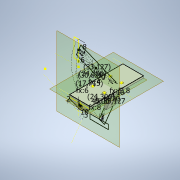
# Autodesk Inventor part: Capping_RotationAnchor
Saved by Autodesk Inventor 2022 (Build 260153000, 153)
## iProperties
Created: 2024-05-05
Part Number: Capping_RotationAnchor
Material: Generic
Document SubType Name: Modeling
Designer: raphael.hauk
Density: 1 g/cm^3
Appearance: Default
Author: raphael.hauk
Autodesk Inventor part; units mm, degrees
ref_plane "YZ Plane" through (0, 0, 0) normal (1, 0, 0) x (0, 1, 0)
ref_plane "XZ Plane" through (0, 0, 0) normal (0, 1, 0) x (-1, 0, 0)
ref_plane "XY Plane" through (0, 0, 0) normal (0, 0, 1) x (1, 0, 0)
sketch "Sketch1" plane through (0, 0, 0) normal (0, 0, 1) x (1, 0, 0)
  line L0 (0, 8) -> (0, -8) projected
  line L1 (0, 8) -> (-4, 8) projected
  line L2 (-4, -8) -> (-4, 8) projected
  line L3 (0, -8) -> (-4, -8) projected
  point P0 (0, 0)
  point P1 (21.25, -8.826)
  constraints: 1 other
sketch "Sketch2" plane through (0, 0, 0) normal (0, 0, 1) x (1, 0, 0)
  line L0 (10, -43.252) -> (26, -43.252)
  line L1 (26, -43.252) -> (26, -47.252)
  line L2 (26, -47.252) -> (10, -47.252)
  line L3 (10, -47.252) -> (10, -43.252)
  line L4 (-4, -8) -> (-4, 8) construction
  line L5 (0, 8) -> (-4, 8) construction
  line L6 (0, 8) -> (0, -8) construction
  line L7 (0, -8) -> (-4, -8) construction
  line L8 (30.626, -12.626) -> (0, 0) construction
  line L9 (18, -43.252) -> (30.626, -12.626) construction
  arc A0 (0, 8) -> (10, -43.252) centre (30.626, -12.626) ccw construction
  line L10 (21.25, -8.826) -> (0, -8.826) construction
  line L11 (1.9057, 4.6226) -> (32.5317, -8.0034)
  line L12 (32.5317, -8.0034) -> (28.7203, -17.2486)
  line L13 (28.7203, -17.2486) -> (-1.9057, -4.6226)
  line L14 (-1.9057, -4.6226) -> (1.9057, 4.6226)
  line L15 (1.9057, 4.6226) -> (28.7203, -17.2486) construction
  line L16 (32.5317, -8.0034) -> (-1.9057, -4.6226) construction
  line L17 (30.626, -12.626) -> (18, -43.252)
  line L18 (18, -43.252) -> (22.6226, -45.1577)
  line L19 (22.6226, -45.1577) -> (35.2486, -14.5317)
  line L20 (35.2486, -14.5317) -> (30.626, -12.626)
  point P0 (23.0031, -31.1163)
  point P1 (12.1357, -5.0031)
  point P2 (15.313, -6.313)
  point P3 (0, 0)
  dimension "d0" = 10
  dimension "d3" = 8
  dimension "d5" = 8
  dimension "d6" = 33.1265
  dimension "d7" = 33.1265
  dimension "d8" = 3.8
  dimension "d9" = 30.626
  dimension "d26" = 20
  dimension "d27" = 20
  dimension "d44" = 10
  dimension "d47" = 5
  constraints: 34 end point, 8 equal length, 8 midpoint, 5 perpendicular, 2 horizontal, 2 point on circle, 2 point on line, 1 centre point, 1 coincident
  measures "d0" distance between parallel lines of L3 L6
  measures "d3" distance of L5.start L8.end
  measures "d5" distance of L0.start L9.start
  measures "d6" distance of L8.start L8.end
  measures "d7" distance of L9.start L8.start
  measures "d8" distance from line of L17.start L10
  measures "d9" distance from line of L6 L17.start
  measures "d26" distance of point (12.136, -5.003) L17.start
  measures "d27" distance of point (23.003, -31.116) L17.start
  measures "d44" distance of L11.end L12.end
  measures "d47" distance of L19.end L17.start
ref_plane "Work Plane1" through (10.248, -8.826, 23.9001) normal (0, -1, 0) x (0, 0, -1)
sketch "Sketch3" plane through (10.248, -8.826, 23.9001) normal (0, -1, 0) x (0, 0, -1)
  circle A0 centre (11.5, 24.802) radius 1.45 construction
  circle A1 centre (26.5, 24.802) radius 1.45 construction
  circle A2 centre (11.5, 14.802) radius 1.45 construction
  circle A3 centre (26.5, 14.802) radius 1.45 construction
  line L0 (-5, 2.002) -> (-5, 21.7091) construction
  line L1 (-5, 10.802) -> (41.5, 10.802)
  line L2 (41.5, 10.802) -> (41.5, 28.802)
  line L3 (41.5, 28.802) -> (-5, 28.802)
  line L4 (-5, 28.802) -> (-5, 10.802)
  line L5 (41.5, 2.002) -> (41.5, 21.7091) construction
  point P0 (23.9001, -10.248)
  dimension "d10" = 4
  dimension "d11" = 4
  constraints: 8 end point, 2 parallel, 2 point on line, 1 horizontal, 1 perpendicular
  measures "d10" distance from line of L3 A0.centre
  measures "d11" distance from line of L1 A2.centre
extrude "Extrusion1" add sketch "Sketch3" along normal blind 2
ref_plane "Work Plane3" through (10.248, -12.826, 23.9001) normal (0, -1, 0) x (1, 0, 0)
sketch "Sketch4" plane through (10.248, -12.826, 23.9001) normal (0, -1, 0) x (1, 0, 0)
  point P0 (-10.248, -23.9001)
  point P1 (14.802, -11.5)
  point P2 (14.802, -26.5)
  point P3 (24.802, -11.5)
  point P4 (24.802, -26.5)
sketch "Sketch5" plane through (21.05, -8.826, 28.9001) normal (0, 0, 1) x (1, 0, 0)
  circle A0 centre (9.576, -3.8) radius 1.5
  line L0 (0, -2) -> (18, -2) projected
  arc A1 (8.4326, -6.5735) -> (12.3686, -4.896) centre (9.576, -3.8) ccw
  line L1 (7.6703, -8.4226) -> (-22.9557, 4.2034) construction
  line L2 (7.6703, -8.4226) -> (-0.7623, -4.9461) construction
  line L3 (-0.7623, -4.9461) -> (0, -3.0971) construction
  line L4 (0, -3.0971) -> (8.4326, -6.5735) construction
  line L5 (8.4326, -6.5735) -> (7.6703, -8.4226) construction
  line L6 (0, -2) -> (0, -3.0971)
  line L7 (0, -3.0971) -> (8.4326, -6.5735)
  line L8 (1.5726, -36.3317) -> (14.1986, -5.7057) construction
  line L9 (14.1986, -5.7057) -> (10.7221, -14.1383) construction
  line L10 (10.7221, -14.1383) -> (8.8731, -13.376) construction
  line L11 (8.8731, -13.376) -> (12.3495, -4.9434) construction
  line L12 (12.3495, -4.9434) -> (14.1986, -5.7057)
  arc A2 (8.4326, -6.5735) -> (12.3495, -4.9434) centre (9.576, -3.8) ccw construction
  line L13 (14.1986, -5.7057) -> (18, -2)
  point P0 (-21.05, 8.826)
  point P1 (12.3495, -4.9434)
  dimension "d21" = 3
  dimension "d46" = 2
  constraints: 22 end point, 5 equal length, 4 perpendicular, 4 point on circle, 4 point on line, 3 centre point, 3 coincident, 1 tangent, 1 vertical
  measures "d21" diameter of A0
  measures "d46" distance between parallel lines of L1 L4
extrude "Extrusion2" add sketch "Sketch5" against normal up to surface (46.5 mm away)
ref_plane "Work Plane5" through (39.05, -8.826, 5.6501) normal (0, 0, -1) x (-1, 0, 0)
sketch "Sketch7" plane through (39.05, -8.826, 5.6501) normal (0, 0, -1) x (-1, 0, 0)
  line L0 (0, -2) -> (5.2779, -14.9628)
  line L1 (5.2779, -14.9628) -> (7.2779, -14.1383)
  line L2 (3.8014, -5.7057) -> (7.2779, -14.1383) construction
  line L3 (0, 0) -> (0, -2) construction
  line L4 (0, -2) -> (3.8014, -5.7057)
  line L5 (7.2779, -14.1383) -> (3.8014, -5.7057)
  point P0 (39.05, 8.826)
  point P1 (0, -2)
  dimension "d51" = 2
  constraints: 8 end point, 1 coincident, 1 collinear, 1 perpendicular
  measures "d51" horizontal distance of L0.end L1.end
extrude "Extrusion3" add sketch "Sketch7" along normal mid plane 8
hole "Hole1" at (25.05, -12.826, -2.5999) at (25.05, -12.826, 12.4001) at (35.05, -12.826, 12.4001) at (35.05, -12.826, -2.5999) direction (0, 1, 0) diameter 2.6 end through all start extended yes counterbore diameter 5.5 counterbore depth 2 clearance for "Socket Head Cap Screw ISO 4762" size "M2.5" standard "ISO"
sketch "Federn" plane through (0, 0, 0) normal (0, 0, 1) x (1, 0, 0)
  line L0 (10, -43.252) -> (26, -43.252) construction
  line L1 (0, 8) -> (0, -8) construction
  line L2 (0, -2) -> (30.626, -12.626) construction
  line L3 (30.626, -12.626) -> (20, -43.252) construction
  arc A0 (0, -2) -> (20, -43.252) centre (30.2135, -12.826) ccw construction
  line L4 (48.9829, -12.826) -> (-20.5476, -12.826) construction
  line L5 (30.626, -12.626) -> (1.3341, -26.8274) construction
  arc A1 (0, -2) -> (20, -43.252) centre (30.2135, -12.826) ccw construction
  line L6 (3.9517, -32.2264) -> (-3.0284, -17.8292) construction
  line L7 (0, -2) -> (17.2743, -19.0992) construction
  line L8 (17.2743, -19.0992) -> (20, -43.252) construction
  line L9 (1.3341, -26.8274) -> (17.2743, -19.0992) construction
  point P0 (0, 0)
  dimension "d28" = 6
  dimension "d33" = 45
  dimension "d39" = 6
  dimension "d40" = 24.306
  dimension "d41" = 17.715
  dimension "d43" = 24.306
  constraints: 14 end point, 7 point on circle, 6 point on line, 2 centre point, 1 equal length, 1 perpendicular, 1 tangent
  measures "d28" distance of L2.start L1.end
  measures "d33" angle of L3 L5
  measures "d39" distance of L6.start L9.start
equation "\"d5\" = d3"
equation "\"d7\" = d6"
equation "\"d27\" = d26"
equation "\"d47\" = 0.5 * d44"
equation "\"d11\" = d10"
equation "\"d39\" = d28"
body "Solid1"
